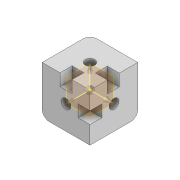
# Autodesk Inventor part: HansKube.stl
Saved by Autodesk Inventor 2021 (Build 250183000, 183)
## iProperties
Created: 2020-12-08
Part Number: HansKube.stl
Material: Generic
Document SubType Name: Modeling
Designer: Alfred Brauner
Density: 1 g/cm^3
Appearance: Default
Author: Alfred Brauner
Autodesk Inventor part; units mm, degrees
ref_plane "YZ Plane" through (0, 0, 0) normal (1, 0, 0) x (0, 1, 0)
ref_plane "XZ Plane" through (0, 0, 0) normal (0, 1, 0) x (-1, 0, 0)
ref_plane "XY Plane" through (0, 0, 0) normal (0, 0, 1) x (1, 0, 0)
sketch "Sketch1" plane through (0, 0, 0) normal (0, 0, 1) x (1, 0, 0)
  line L0 (-10, 10) -> (10, 10)
  line L1 (10, 10) -> (10, -10)
  line L2 (10, -10) -> (-10, -10)
  line L3 (-10, -10) -> (-10, 10)
  line L4 (-10, 10) -> (10, -10) construction
  line L5 (10, 10) -> (-10, -10) construction
  point P0 (0, 0)
  dimension "d0" = 20
  dimension "d1" = 20
  constraints: 12 end point, 2 midpoint, 2 parallel, 1 horizontal, 1 perpendicular
  measures "d0" distance of L1.end L2.end
  measures "d1" distance of L0.end L1.end
extrude "Extrusion1" add sketch "Sketch1" along normal mid plane 20
sketch "Sketch2" plane through (0, 0, 10) normal (0, 0, 1) x (1, 0, 0)
  line L0 (10, 10) -> (-10, 10) projected
  line L1 (-2.5, 10) -> (2.5, 10)
  line L2 (2.5, 10) -> (2.5, 5)
  line L3 (2.5, 5) -> (-2.5, 5)
  line L4 (-2.5, 5) -> (-2.5, 10)
  line L5 (-10, 10) -> (-10, -10) projected
  line L6 (10, -10) -> (10, 10) projected
  line L7 (10, 2.5) -> (5, 2.5)
  line L8 (5, 2.5) -> (5, -2.5)
  line L9 (5, -2.5) -> (10, -2.5)
  line L10 (10, -2.5) -> (10, 2.5)
  point P0 (0, 0)
  dimension "d4" = 5
  dimension "d5" = 5
  dimension "d6" = 7.5
  dimension "d7" = 5
  dimension "d8" = 5
  dimension "d9" = 7.5
  constraints: 16 end point, 4 parallel, 2 horizontal, 2 perpendicular, 2 point on line
  measures "d4" distance of L2.end L3.end
  measures "d5" distance of L1.end L2.end
  measures "d6" distance between parallel lines of L4 L5
  measures "d7" distance between parallel lines of L7 L9
  measures "d8" distance between parallel lines of L8 L6
  measures "d9" distance between parallel lines of L7 L0
extrude "Extrusion2" cut sketch "Sketch2" against normal blind 5
sketch "Sketch3" plane through (10, -10, -10) normal (1, 0, 0) x (0, 0, -1)
  line L0 (0, 20) -> (-20, 20) projected
  line L1 (-12.7592, 20) -> (-7.7592, 20)
  line L2 (-7.7592, 20) -> (-7.7592, 15)
  line L3 (-7.7592, 15) -> (-12.7592, 15)
  line L4 (-12.7592, 15) -> (-12.7592, 20)
  point P0 (-10, 10)
  dimension "d12" = 5
  dimension "d13" = 5
  constraints: 8 end point, 2 parallel, 1 horizontal, 1 perpendicular, 1 point on line
  measures "d12" distance of L2.end L3.end
  measures "d13" distance between parallel lines of L0 L3
extrude "Extrusion3" cut sketch "Sketch3" against normal blind 5
sketch "Sketch8" plane through (-10, -10, 10) normal (-1, 0, 0) x (0, 0, 1)
  circle A0 centre (-10, 10) radius 2.3529
  constraints: 1 centre point, 1 coincident
sketch "Sketch9" plane through (-10, -10, 10) normal (0, -1, 0) x (1, 0, 0)
  circle A0 centre (10, -10) radius 2.6586
  constraints: 1 centre point, 1 coincident
sketch "Sketch10" plane through (0, 0, -10) normal (0, 0, -1) x (-1, 0, 0)
  circle A0 centre (0, 0) radius 2.2697
  constraints: 1 centre point, 1 coincident
hole "Hole3" at (0, -10, 0) direction (0, 1, 0) diameter 4 depth 29.3 tip angle 118 counterbore diameter 8 counterbore depth 17.5
hole "Hole4" at (0, 0, -10) direction (0, 0, 1) diameter 4 depth 29.3 tip angle 118 counterbore diameter 8 counterbore depth 17.5
hole "Hole5" at (-10, 0, 0) direction (1, 0, 0) diameter 4 depth 29.3 tip angle 118 counterbore diameter 8 counterbore depth 17.5
fillet "Fillet2" radius 3 3 edges at (0, -10, -10) (-10, -10, 0) (-10, 0, -10)
body "Solid1"
